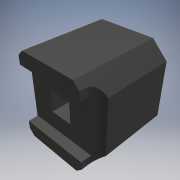
# Autodesk Inventor part: Housing male header - single
Saved by Autodesk Inventor 2017 (Build 210142000, 142)
## iProperties
Created: 2017-09-07
Part Number: Housing male header - single
Material: ABS Plastic
Document SubType Name: Modeling
Designer: denoqs
Density: 1.06 g/cm^3
Appearance: Smooth - White(1)
Author: denoqs
Autodesk Inventor part; units mm, degrees
ref_plane "YZ Plane" through (0, 0, 0) normal (1, 0, 0) x (0, 1, 0)
ref_plane "XY Plane" through (0, 0, 0) normal (0, 0, 1) x (1, 0, 0)
sketch "Sketch1" plane through (0, 0, 0) normal (0, 1, 0) x (-1, 0, 0)
  line L0 (1.27, -1.27) -> (-1.27, -1.27)
  line L1 (-1.27, -1.27) -> (-1.27, 1.27)
  line L2 (-1.27, 1.27) -> (1.27, 1.27)
  line L3 (1.27, 1.27) -> (1.27, -1.27)
  point P0 (0, 0)
  point P1 (0, -1.27)
  point P2 (-1.27, 0)
  dimension "d0" = 2.54
  dimension "d1" = 2.54
  constraints: 8 end point, 2 midpoint, 2 parallel, 1 horizontal, 1 horizontal alignment, 1 perpendicular, 1 vertical alignment
  measures "d0" distance of L0.start L0.end
  measures "d1" distance of L0.end L1.end
extrude "Extrusion1" add sketch "Sketch1" along normal blind 2.54
sketch "Sketch2" plane through (0, 2.54, 0) normal (0, 1, 0) x (1, 0, 0)
  line L0 (-0.325, 0.325) -> (0.325, 0.325)
  line L1 (0.325, 0.325) -> (0.325, -0.325)
  line L2 (0.325, -0.325) -> (-0.325, -0.325)
  line L3 (-0.325, -0.325) -> (-0.325, 0.325)
  point P0 (0, 0)
  point P1 (0, 0.325)
  point P2 (0.325, 0)
  dimension "d4" = 0.65
  dimension "d5" = 0.65
  constraints: 8 end point, 2 midpoint, 2 parallel, 1 horizontal, 1 horizontal alignment, 1 perpendicular, 1 vertical alignment
  measures "d4" distance of L1.end L2.end
  measures "d5" distance of L0.end L1.end
extrude "Extrusion2" cut sketch "Sketch2" against normal up to next
chamfer "Chamfer1" distance 0.45 angle 45 4 edges at (1.27, 1.27, 1.27) (-1.27, 1.27, 1.27) (1.27, 1.27, -1.27) (-1.27, 1.27, -1.27)
sketch "Sketch3" plane through (0, 0, 0) normal (1, 0, 0) x (0, 1, 0)
  line L0 (0, -0.82) -> (2.54, -0.82) projected
  line L1 (0, 0.82) -> (0, -0.82) projected
  line L2 (2.54, 0.82) -> (0, 0.82) projected
  line L3 (2.54, -0.82) -> (2.54, 0.82) projected
  line L4 (2.54, 1.27) -> (2.54, 0.82) projected
  line L5 (2.54, 0.82) -> (0, 0.82) projected
  line L6 (0, 0.82) -> (0, 1.27) projected
  line L7 (0, 1.27) -> (2.54, 1.27) projected
  line L8 (2.54, -0.82) -> (2.54, -1.27) projected
  line L9 (2.54, -1.27) -> (0, -1.27) projected
  line L10 (0, -1.27) -> (0, -0.82) projected
  line L11 (0, -0.82) -> (2.54, -0.82) projected
  line L12 (0, 0.82) -> (0, -0.82) projected
  line L13 (0, 0.85) -> (0.3, 0.85)
  line L14 (0.3, 0.85) -> (0.3, -0.85)
  line L15 (0.3, -0.85) -> (0, -0.85)
  line L16 (0, -0.85) -> (0, 0.85)
  point P0 (0, 0)
  point P1 (0.3, 0)
  dimension "d11" = 0.3
  dimension "d16" = 1.7
  constraints: 8 end point, 2 parallel, 1 horizontal, 1 horizontal alignment, 1 midpoint, 1 perpendicular, 1 point on line
  measures "d11" distance of L14.end L15.end
  measures "d16" distance of L13.end L14.end
extrude "Extrusion3" cut sketch "Sketch3" along normal mid plane 2.54 contours L1 L2 L14 L0 | L0 L14 L15 L10 | L6 L13 L14 L2
sketch "Sketch5" plane through (0, 0, 0) normal (0, 0, 1) x (1, 0, 0)
  line L0 (-1.27, 0.3) -> (-1.27, 2.54) projected
  line L1 (-1.27, 2.54) -> (-1.27, 0.3) projected
  line L2 (-1.27, 0.3) -> (-1.27, 2.54) projected
  line L3 (-1.24, 0.3) -> (-1.27, 0.3) projected
  line L4 (-1.27, 0.3) -> (-1.27, 2.54) projected
  line L5 (-1.27, 2.54) -> (-0.82, 2.54) projected
  line L6 (-0.82, 2.54) -> (-0.82, 0) projected
  line L7 (-0.82, 0) -> (-1.24, 0) projected
  line L8 (-1.24, 0) -> (-1.24, 0.3) projected
  line L9 (-0.9925, 0) -> (-0.9925, 0.1729)
  arc A0 (-0.9925, 0.1729) -> (-1.27, 0.5088) centre (-1.3346, 0.1729) ccw
  point P0 (0, 0)
  constraints: 2 end point, 2 point on circle, 2 point on line, 1 centre point, 1 tangent, 1 vertical
extrude "Extrusion5" cut sketch "Sketch5" along normal mid plane 2.54 contours L0 A0 L9 L7 L8 L3
mirror "Mirror2" about plane through (0, 0, 0) normal (1, 0, 0) of "Extrusion5"
ref_plane "Work Plane1" through (0, -2.54, 0) normal (0, 1, 0) x (-1, 0, 0)
sketch "Sketch6" plane through (0, -2.54, 0) normal (0, 1, 0) x (-1, 0, 0)
  line L0 (0.325, -0.325) -> (-0.325, -0.325) projected
  line L1 (0.325, 0.325) -> (0.325, -0.325) projected
  line L2 (-0.325, 0.325) -> (0.325, 0.325) projected
  line L3 (-0.325, -0.325) -> (-0.325, 0.325) projected
  point P0 (0, 0)
equation "\"d1\" = d0"
equation "\"d4\" = d5"
body "Solid1"
